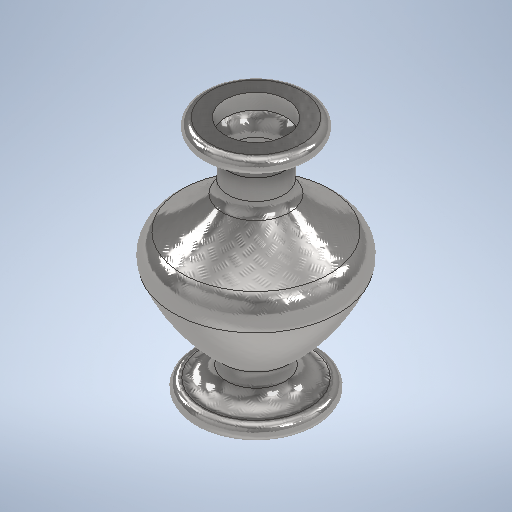
# Autodesk Inventor part: cad@66
Saved by Autodesk Inventor 2025.2 (Build 292293000, 293)
## iProperties
Created: 2025-04-22
Part Number: cad@66
Material: Generic
Document SubType Name: Modeling
Designer: spars
Density: 1 g/cm^3
Appearance: Diamond Plate
Author: spars
Autodesk Inventor part; units mm, degrees
ref_plane "YZ Plane" through (0, 0, 0) normal (1, 0, 0) x (0, 1, 0)
ref_plane "XZ Plane" through (0, 0, 0) normal (0, 1, 0) x (-1, 0, 0)
ref_plane "XY Plane" through (0, 0, 0) normal (0, 0, 1) x (1, 0, 0)
sketch "Sketch1" plane through (0, 0, 0) normal (0, 0, 1) x (1, 0, 0)
  line L0 (-263.2137, 47.6556) -> (-59.7844, 47.6556) construction
  line L1 (-59.7844, 47.6556) -> (-59.7844, -127.6195) construction
  line L2 (-59.7844, -127.6195) -> (-263.2137, -127.6195) construction
  line L3 (-263.2137, -127.6195) -> (-263.2137, 47.6556) construction
  line L4 (-20.7845, 161.3393) -> (-30.7845, 161.3393)
  arc A0 (-30.7845, 161.3393) -> (-30.7845, 151.3393) centre (-30.7845, 156.3393) ccw
  arc A1 (-19.6579, 17.5616) -> (-21.7885, 28.5295) centre (-27.65, 21.7) ccw
  arc A2 (-35.2927, 9.9162) -> (-36.2044, 0) centre (-36.2044, 5) ccw
  arc A3 (-49.4635, 94.9438) -> (-55.7151, 75.2482) centre (-40.945, 81.4) ccw
  arc A4 (-55.7151, 75.2482) -> (-21.7885, 28.5295) centre (59.4915, 123.2322) ccw
  arc A5 (-35.2927, 9.9162) -> (-19.6579, 17.5616) centre (-32.629, 24.2782) ccw
  arc A6 (-18.7845, 139.3393) -> (-30.7845, 151.3393) centre (-30.7845, 139.3393) ccw
  line L5 (-18.7845, 139.3393) -> (-18.7845, 125.6393)
  arc A7 (-22.3796, 117.0743) -> (-18.7845, 125.6393) centre (-30.7845, 125.6393) ccw
  arc A8 (-49.4635, 94.9438) -> (-21.7885, 117.6975) centre (-124.9562, 214.9723) ccw
  line L6 (0, 0) -> (0, 197.1464)
  line L7 (0, 0) -> (0, -39.9819)
  line L8 (-36.2044, 0) -> (0, 0)
  line L9 (0, 4) -> (-36.2044, 4)
  arc A9 (-36.0221, 5.9832) -> (-36.2044, 4) centre (-36.2044, 5) ccw
  arc A10 (-36.0221, 5.9832) -> (-16.1058, 15.7223) centre (-32.629, 24.2782) ccw
  arc A11 (-16.1058, 15.7223) -> (-19.1833, 31.5649) centre (-27.65, 21.7) ccw
  arc A12 (-52.0226, 76.7862) -> (-19.1833, 31.5649) centre (59.4915, 123.2322) ccw
  arc A13 (-47.3339, 91.5579) -> (-52.0226, 76.7862) centre (-40.945, 81.4) ccw
  arc A14 (-47.3339, 91.5579) -> (-18.8781, 114.9534) centre (-124.9562, 214.9723) ccw
  arc A15 (-14.7845, 139.3393) -> (-20.2015, 151.3393) centre (-30.7845, 139.3393) ccw
  line L10 (-14.7845, 139.3393) -> (-14.7845, 125.6393)
  arc A16 (-19.578, 114.2193) -> (-14.7845, 125.6393) centre (-30.7845, 125.6393) ccw
  line L11 (-20.7845, 161.3393) -> (-20.2015, 151.3393)
  line L12 (0, 4) -> (0, 0)
  point P0 (-0.7845, 155.0151)
  point P1 (34.2155, 155.0151)
  point P2 (-35.7845, 156.3393)
  point P3 (-19.5283, 114.2683)
  dimension "d12" = 5
  dimension "d21" = 18
  dimension "d24" = 10
  dimension "d25" = 32
  dimension "d26" = 59.7
  dimension "d27" = 124.8
  dimension "d32" = 24
  dimension "d33" = 13.7
  dimension "d34" = 24
  dimension "d36" = 16.7
  dimension "d39" = 4
  constraints: 37 point on circle, 18 end point, 17 centre point, 9 tangent, 3 vertical, 1 collinear, 1 horizontal, 9 other
  measures "d12" radius of A0
  measures "d21" diameter of A1
  measures "d24" diameter of A2
  measures "d25" diameter of A3
  measures "d26" vertical distance of A1.centre A3.centre
  measures "d27" radius of A4
  measures "d32" diameter of A6
  measures "d33" distance of L5.start L5.end
  measures "d34" diameter of A7
  measures "d36" vertical distance of A2.centre A1.centre
  measures "d39" distance between parallel lines of L8 L9
revolve "Revolution1" add sketch "Sketch1" angle 360 about axis through (0, 0, 0) along (0, 1, 0) contours L11 A15 L10 A16 A14 A13 A12 A11 A10 A9 L9 L6 L8 A2 A5 A1 A4 A3 A8 A7 L5 A6 A0 L4
body "Solid1"
